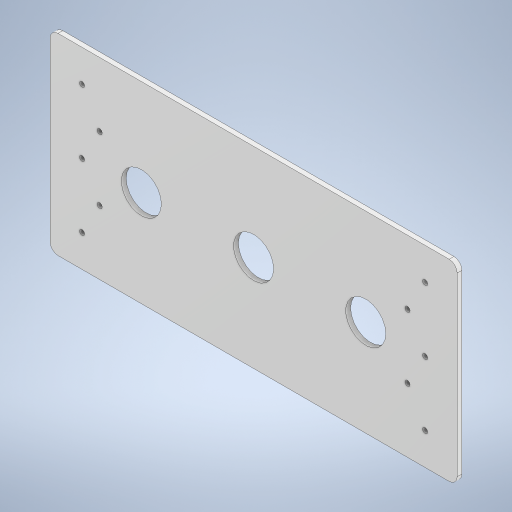
# Autodesk Inventor part: BP_BOX-Front-120
Saved by Autodesk Inventor 2024.3 (Build 283343000, 343)
## iProperties
Created: 2025-04-19
Part Number: BP_BOX-Front-120
Material: アセタール樹脂、白
Document SubType Name: Modeling
Designer: ngt-a
Density: 1.425 g/cm^3
Appearance: 滑らか - 白
Mass: 67.1611 g
Surface Area: 355.524 cm^2
Volume: 51.268 cm^3
Author: ngt-a
Autodesk Inventor part; units mm, degrees
ref_plane "YZ Plane" through (0, 0, 0) normal (1, 0, 0) x (0, 1, 0)
ref_plane "XZ Plane" through (0, 0, 0) normal (0, 1, 0) x (-1, 0, 0)
ref_plane "XY Plane" through (0, 0, 0) normal (0, 0, 1) x (1, 0, 0)
sketch "スケッチ1" plane through (0, 0, 0) normal (0, 1, 0) x (-1, 0, 0)
  line L0 (130, 1.5) -> (-130, 1.5)
  line L1 (-130, 1.5) -> (-130, -1.5)
  line L2 (-130, -1.5) -> (130, -1.5)
  line L3 (130, -1.5) -> (130, 1.5)
  line L4 (130, 1.5) -> (-130, -1.5) construction
  line L5 (-130, 1.5) -> (130, -1.5) construction
  point P0 (0, 0)
  dimension "d0" = 260
  dimension "d1" = 3
  constraints: 12 end point, 2 midpoint, 2 parallel, 1 horizontal, 1 perpendicular
  measures "d0" distance of L1.end L2.end
  measures "d1" distance of L2.end L0.start
extrude "押し出し1" add sketch "スケッチ1" along normal blind 120
sketch "スケッチ3" plane through (-130, 0, 1.5) normal (0, 0, 1) x (1, 0, 0)
  circle A0 centre (60, 60) radius 12.5
  circle A1 centre (130, 60) radius 12.5
  circle A2 centre (200, 60) radius 12.5
  line L0 (0, 0) -> (0, 120) projected
  line L1 (260, 0) -> (260, 120) projected
  point P0 (130, 0)
  point P1 (0, 60)
  point P2 (260, 60)
  dimension "d10" = 25
  dimension "d11" = 25
  dimension "d12" = 25
  dimension "d15" = 60
  dimension "d16" = 60
  dimension "d18" = 0
  dimension "d21" = 0
  dimension "d71" = 0
  dimension "d72" = 70
  constraints: 3 centre point, 2 midpoint
  measures "d10" diameter of A0
  measures "d11" diameter of A2
  measures "d12" diameter of A1
  measures "d15" distance from line of A0.centre L0
  measures "d16" distance from line of L1 A2.centre
  measures "d18" vertical distance of point (0, 60) A0.centre
  measures "d21" vertical distance of point (260, 60) A2.centre
  measures "d71" vertical distance of A1.centre A0.centre
  measures "d72" distance of A2.centre A1.centre
extrude "押し出し3" cut sketch "スケッチ3" against normal through all
sketch "スケッチ5" plane through (130, 0, -1.5) normal (0, 0, -1) x (-1, 0, 0)
  line L0 (0, 0) -> (260, 0) projected
  line L1 (0, 120) -> (3, 120)
  line L2 (3, 120) -> (3, 0)
  line L3 (3, 0) -> (0, 0)
  line L4 (0, 0) -> (0, 120)
  line L5 (0, 105) -> (3, 105)
  line L6 (3, 105) -> (3, 15)
  line L7 (3, 15) -> (0, 15)
  line L8 (0, 15) -> (0, 105)
  line L9 (0, 120) -> (260, 120) projected
  line L10 (130, 120) -> (130, 0)
  line L11 (260, 0) -> (0, 0)
  line L12 (260, 120) -> (257, 120)
  line L13 (257, 120) -> (257, 0)
  line L14 (260, 0) -> (260, 120)
  line L15 (260, 105) -> (257, 105)
  line L16 (257, 15) -> (260, 15)
  point P0 (1.5, 105)
  point P1 (1.5, 120)
  point P2 (1.5, 15)
  point P3 (1.5, 0)
  point P4 (258.5, 15)
  point P5 (257, 0)
  point P6 (257, 120)
  point P7 (0, 15)
  point P8 (3, 105)
  dimension "d22" = 3
  dimension "d23" = 15
  dimension "d24" = 15
  constraints: 30 end point, 10 symmetric about line, 6 point on line, 5 midpoint, 4 parallel, 3 perpendicular, 2 horizontal
  measures "d22" distance between parallel lines of L2 L4
  measures "d23" distance of point (1.5, 105) point (1.5, 120)
  measures "d24" distance of point (1.5, 15) point (1.5, 0)
extrude "押し出し4" cut sketch "スケッチ5" against normal through all contours L4 L7 L2 L0 | L4 L5 L2 L7 | L4 L1 L2 L5 | L13 L16 L14 L0 | L13 L15 L14 L16 | L9 L14 L15 L13
sketch "スケッチ8" plane through (-127, 0, 1.5) normal (0, 0, 1) x (1, 0, 0)
  circle A0 centre (20, 100) radius 1.6
  circle A1 centre (20, 20) radius 1.6
  line L0 (0, 120) -> (0, 0) projected
  line L1 (0, 120) -> (254, 120) projected
  line L2 (0, 0) -> (254, 0) projected
  line L3 (127, 120) -> (127, 0)
  circle A2 centre (234, 100) radius 1.6
  circle A3 centre (234, 20) radius 1.6
  circle A4 centre (20, 60) radius 1.6
  circle A5 centre (234, 60) radius 1.6
  dimension "d31" = 20
  dimension "d32" = 20
  dimension "d33" = 20
  dimension "d34" = 20
  dimension "d35" = 3.2
  dimension "d36" = 3.2
  dimension "d73" = 3.2
  dimension "d74" = 40
  dimension "d75" = 20
  constraints: 6 centre point, 3 symmetric about line, 2 end point, 1 midpoint, 1 vertical, 3 other
  measures "d31" distance from line of A0.centre L0
  measures "d32" distance from line of A0.centre L1
  measures "d33" distance from line of A1.centre L0
  measures "d34" distance from line of L2 A1.centre
  measures "d35" diameter of A0
  measures "d36" diameter of A1
  measures "d73" diameter of A4
  measures "d74" distance of A1.centre A4.centre
  measures "d75" distance from line of L0 A4.centre
extrude "押し出し7" cut sketch "スケッチ8" against normal through all contours A0 | A1 | A2 | A3 | A4 | A5
fillet "フィレット1" radius 5 4 edges at (-127, 120, 0) (-127, 0, 0) (127, 120, 0) (127, 0, 0)
sketch "スケッチ13" plane through (-122, 0, 1.5) normal (0, 0, 1) x (1, 0, 0)
  line L0 (244, 120) -> (0, 120) projected
  line L1 (122, 120) -> (122, 0)
  circle A0 centre (15, 110) radius 1.6 projected
  circle A1 centre (15, 10) radius 1.6 projected
  circle A2 centre (15, 60) radius 1.6 projected
  circle A3 centre (122, 60) radius 12.5 projected
  line L2 (122, 60) -> (122, 88.3789)
  point P0 (26, 80)
  point P1 (26, 40)
  point P2 (218, 80)
  point P3 (218, 40)
  dimension "d76" = 11
  dimension "d77" = 40
  dimension "d78" = 20
  dimension "d79" = 11
  constraints: 4 end point, 2 symmetric about line, 2 vertical, 1 midpoint
  measures "d76" horizontal distance of A0.centre point (26, 80)
  measures "d77" distance of point (26, 40) point (26, 80)
  measures "d78" vertical distance of A2.centre point (26, 40)
  measures "d79" horizontal distance of A1.centre point (26, 40)
hole "穴1" at (-96, 80, 1.5) at (-96, 40, 1.5) at (96, 40, 1.5) at (96, 80, 1.5) direction (0, 0, -1) diameter 3.2 end through all
equation "\"d36\" = d35"
equation "\"d73\" = d35"
equation "\"d78\" = 0.5 * d77"
